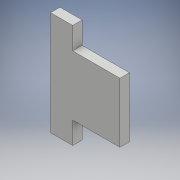
# Autodesk Inventor part: k2_dist
Saved by Autodesk Inventor 2017 (Build 210142000, 142)
## iProperties
Created: 2017-02-16
Part Number: k2_dist
Material: Generic
Document SubType Name: Modeling
Designer: herman
Density: 1 g/cm^3
Appearance: Default
Author: herman
Autodesk Inventor part; units mm, degrees
ref_plane "YZ Plane" through (0, 0, 0) normal (1, 0, 0) x (0, 1, 0)
ref_plane "XZ Plane" through (0, 0, 0) normal (0, 1, 0) x (-1, 0, 0)
ref_plane "XY Plane" through (0, 0, 0) normal (0, 0, 1) x (1, 0, 0)
sketch "Sketch3" plane through (0, 0, 0) normal (0, 1, 0) x (-1, 0, 0)
  line L0 (-9.6464, 12.476) -> (5.3536, 12.476)
  line L1 (5.3536, 12.476) -> (5.3536, 19.476)
  line L2 (5.3536, 19.476) -> (12.3536, 19.476)
  line L3 (12.3536, 19.476) -> (12.3536, -13.524)
  line L4 (12.3536, -13.524) -> (5.3536, -13.524)
  line L5 (5.3536, -13.524) -> (5.3536, -6.524)
  line L6 (5.3536, -6.524) -> (-9.6464, -6.524)
  line L7 (-9.6464, -6.524) -> (-9.6464, 12.476)
  point P0 (0, 0)
  dimension "d13" = 33
  dimension "d14" = 19
  dimension "d15" = 15
  dimension "d16" = 7
  constraints: 16 end point, 6 perpendicular, 2 point on line, 1 collinear, 1 horizontal
  measures "d13" distance of L2.end L3.end
  measures "d14" distance of L6.end L0.start
  measures "d15" distance of L0.start L0.end
  measures "d16" distance of L1.end L2.end
extrude "Extrusion3" add sketch "Sketch3" along normal blind 3
body "Solid2"
